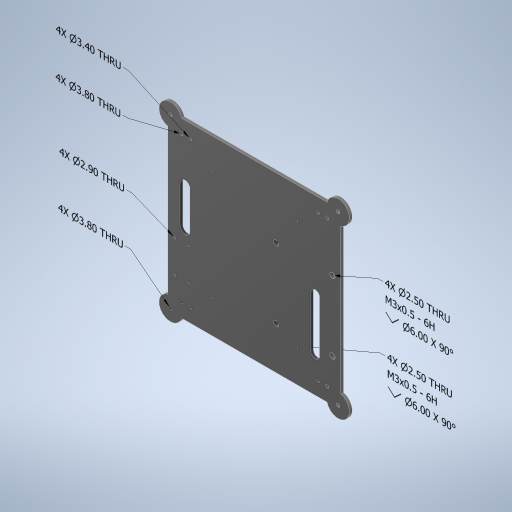
# Autodesk Inventor part: payload_bay_b210_inventor
Saved by Autodesk Inventor 2023.2 (Build 272271030, 271C)
## iProperties
Created: 2023-02-11
Part Number: payload_bay_b210_inventor
Material: ABS Plastic
Document SubType Name: Modeling
Designer: makhi
Density: 1.06 g/cm^3
Appearance: Smooth - White
Author: makhi
Autodesk Inventor part; units mm, degrees
ref_plane "YZ Plane" through (0, 0, 0) normal (1, 0, 0) x (0, 1, 0)
ref_plane "XZ Plane" through (0, 0, 0) normal (0, 1, 0) x (-1, 0, 0)
ref_plane "XY Plane" through (0, 0, 0) normal (0, 0, 1) x (1, 0, 0)
sketch "Board outline" plane through (0, 0, 0) normal (0, 0, 1) x (1, 0, 0)
  line L0 (-95, 95) -> (95, 95)
  line L1 (95, 95) -> (95, -95)
  line L2 (95, -95) -> (-95, -95)
  line L3 (-95, -95) -> (-95, 95)
  circle A0 centre (92, 92) radius 12.5002
  circle A1 centre (-92, 92) radius 12.5002
  circle A2 centre (92, -92) radius 12.5002
  circle A3 centre (-92, -92) radius 12.5002
  point P0 (-79.8652, -95)
  point P1 (79.8652, -95)
  point P2 (95, -79.8651)
  point P3 (95, 79.8651)
  point P4 (79.8652, 95)
  point P5 (-79.8652, 95)
  point P6 (-95, 79.8651)
  point P7 (-95, -79.8651)
  constraints: 8 end point, 4 centre point, 2 parallel, 1 horizontal, 1 perpendicular
extrude "Extrusion1" add sketch "Board outline" along normal blind 3
sketch "Level 2-3 #6 standoff holes" plane through (0, 0, 3) normal (0, 0, 1) x (1, 0, 0)
  circle A0 centre (92, 92) radius 1.8984
  circle A1 centre (-92, -92) radius 1.8984
  circle A2 centre (-92, 92) radius 1.8984
  circle A3 centre (92, -92) radius 1.8984
  constraints: 4 centre point
sketch "B210 countersink holes" plane through (0, 0, 0) normal (0, 0, 1) x (1, 0, 0)
  circle A0 centre (46.8, 60) radius 1.4998
  circle A1 centre (-46.8, 60) radius 1.4998
  circle A2 centre (46.8, -60) radius 1.4998
  circle A3 centre (-46.8, -60) radius 1.4998
  constraints: 4 centre point
sketch "OpenUPS mount holes" plane through (0, 0, 3) normal (0, 0, 1) x (1, 0, 0)
  circle A0 centre (85.86, 28.3) radius 1.5002
  circle A1 centre (85.86, -48.3) radius 1.5002
  circle A2 centre (24.14, 28.3) radius 1.5002
  circle A3 centre (24.14, -48.3) radius 1.5002
  constraints: 4 centre point
hole "Hole2" at (46.8, 60, 0) at (-46.8, 60, 0) at (-46.8, -60, 0) at (46.8, -60, 0) direction (0, 0, 1) diameter 2.459 end through all countersink diameter 6 countersink angle 90 thread size "M3x0.5" class "6H" standard "ISO Metric profile"
hole "Hole3" at (24.14, 28.3, 3) at (85.86, 28.3, 3) at (85.86, -48.3, 3) at (24.14, -48.3, 3) direction (0, 0, -1) diameter 2.459 end through all countersink diameter 6 countersink angle 90 thread size "M3x0.5" class "6H" standard "ISO Metric profile"
sketch "Level 1-2 #6 standoff holes" plane through (0, 0, 3) normal (0, 0, 1) x (1, 0, 0)
  circle A0 centre (80, 80) radius 1.8983
  circle A1 centre (-80, 80) radius 1.8983
  circle A2 centre (80, -80) radius 1.8983
  circle A3 centre (-80, -80) radius 1.8983
  constraints: 4 centre point
sketch "Level 1 M3 standoff holes" plane through (0, 0, 3) normal (0, 0, 1) x (1, 0, 0)
  circle A0 centre (70, 80) radius 1.4998
  circle A1 centre (-70, 80) radius 1.4998
  circle A2 centre (-70, -80) radius 1.4998
  circle A3 centre (70, -80) radius 1.4998
  constraints: 4 centre point
hole "Hole4" at (-70, 80, 3) at (70, 80, 3) at (70, -80, 3) at (-70, -80, 3) direction (0, 0, -1) diameter 3.4 end through all clearance for "Flat Head Machine Screw" size "M3" standard "Ansi Metric M Profile"
hole "Hole5" at (-80, 80, 3) at (80, 80, 3) at (80, -80, 3) at (-80, -80, 3) direction (0, 0, -1) diameter 3.797 end through all clearance for "Flat Head Machine Screw (82)" size "#6" standard "Ansi Unified Screw Threads"
hole "Hole6" at (-92, -92, 3) at (92, -92, 3) at (92, 92, 3) at (-92, 92, 3) direction (0, 0, -1) diameter 3.797 end through all clearance for "Flat Head Machine Screw (82)" size "#6" standard "Ansi Unified Screw Threads"
sketch "Cable cutouts" plane through (0, 0, 3) normal (0, 0, 1) x (1, 0, 0)
  line L0 (-76.0002, 58.0001) -> (-75.9998, 58.0001)
  line L1 (-75.9998, 5.9999) -> (-76.0002, 5.9999)
  arc A0 (-81.5002, -8.5001) -> (-76.0002, -14.0001) centre (-76.0002, -8.5001) ccw
  arc A1 (-70.4998, 32.5001) -> (-75.9998, 38.0001) centre (-75.9998, 32.5001) ccw
  arc A2 (-76.0002, 38.0001) -> (-81.5002, 32.5001) centre (-76.0002, 32.5001) ccw
  line L2 (-81.5002, -8.5001) -> (-81.5002, 32.5001)
  line L3 (-75.9998, -14.0001) -> (-76.0002, -14.0001)
  line L4 (-70.4998, 32.5001) -> (-70.4998, -8.5001)
  line L5 (-76.0002, 38.0001) -> (-75.9998, 38.0001)
  arc A3 (-75.9998, -14.0001) -> (-70.4998, -8.5001) centre (-75.9998, -8.5001) ccw
  line L6 (66.8002, 5.2998) -> (66.7998, 5.2998)
  line L7 (71.7998, 0.2998) -> (71.7998, -55.6998)
  line L8 (66.7998, -60.6998) -> (66.8002, -60.6998)
  line L9 (61.8002, -55.6998) -> (61.8002, 0.2998)
  arc A4 (66.8002, 5.2998) -> (61.8002, 0.2998) centre (66.8002, 0.2998) ccw
  arc A5 (71.7998, 0.2998) -> (66.7998, 5.2998) centre (66.7998, 0.2998) ccw
  arc A6 (61.8002, -55.6998) -> (66.8002, -60.6998) centre (66.8002, -55.6998) ccw
  arc A7 (66.7998, -60.6998) -> (71.7998, -55.6998) centre (66.7998, -55.6998) ccw
  point P0 (66.8, -27.7)
  point P1 (66.8, 5.2998)
  dimension "d58" = 5.5
  dimension "d60" = 5
  constraints: 20 end point, 16 point on circle, 16 tangent, 8 centre point, 6 equal radius, 5 parallel, 3 horizontal, 2 perpendicular
  measures "d58" radius of A2
  measures "d60" radius of A4
extrude "Extrusion2" cut sketch "Cable cutouts" against normal blind 3
sketch "5v Pololu regulator mount holes" plane through (0, 0, 3) normal (0, 0, 1) x (1, 0, 0)
  circle A0 centre (-72.5, -22.25) radius 1.2501
  circle A1 centre (-87.5, -22.25) radius 1.2501
  circle A2 centre (-72.5, -57.75) radius 1.2501
  circle A3 centre (-87.5, -57.75) radius 1.2501
  constraints: 4 centre point
hole "Hole7" at (-87.5, -22.25, 3) at (-72.5, -22.25, 3) at (-72.5, -57.75, 3) at (-87.5, -57.75, 3) direction (0, 0, -1) diameter 2.9 end through all clearance for "Flat Head Machine Screw" size "M2.5" standard "Ansi Metric M Profile"
body "Solid1"
